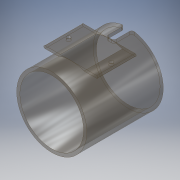
# Autodesk Inventor part: Propeller Shroud
Saved by Autodesk Inventor 2019 (Build 230136000, 136)
## iProperties
Created: 2019-02-08
Part Number: Propeller Shroud
Material: ABS Plastic
Document SubType Name: Modeling
Designer: User
Density: 1.06 g/cm^3
Appearance: Dark Bronze Reflective
Mass: 159.619 g
Surface Area: 631.201 cm^2
Volume: 150.584 cm^3
Author: User
Autodesk Inventor part; units mm, degrees
ref_plane "YZ Plane" through (0, 0, 0) normal (1, 0, 0) x (0, 1, 0)
ref_plane "XZ Plane" through (0, 0, 0) normal (0, 1, 0) x (-1, 0, 0)
ref_plane "XY Plane" through (0, 0, 0) normal (0, 0, 1) x (1, 0, 0)
sketch "Sketch1" plane through (0, 0, 0) normal (0, 0, 1) x (1, 0, 0)
  arc A0 (-20.5913, 51) -> (20.5913, 51) centre (0, 0) ccw
  circle A1 centre (0, 0) radius 50
  line L0 (-40.5, 55) -> (40.5, 55)
  arc A2 (-40.5, 55) -> (-40.5, 51) centre (-40.5, 53) ccw
  arc A3 (40.5, 51) -> (40.5, 55) centre (40.5, 53) ccw
  line L1 (40.5, 51) -> (19.5959, 51)
  line L2 (40.5, 51) -> (19.5959, 51)
  line L3 (40.5, 51) -> (19.5959, 51)
  line L4 (19.5959, 51) -> (-40.5, 51)
  line L5 (0, 51) -> (0, 50)
  dimension "d0" = 110
  dimension "d1" = 100
  constraints: 12 end point, 6 point on circle, 4 centre point, 3 point on line, 2 coincident, 1 horizontal, 1 vertical
  measures "d0" diameter of A0
  measures "d1" diameter of A1
extrude "Extrusion1" add sketch "Sketch1" against normal blind 120
sketch "Sketch2" plane through (0, 0, 0) normal (0, 0, 1) x (1, 0, 0)
  circle A0 centre (0, 0) radius 50 projected
  line L0 (-40.5, 51) -> (-20.5913, 51) projected
  arc A1 (-20.5913, 51) -> (20.5913, 51) centre (0, 0) ccw projected
  line L1 (20.5913, 51) -> (40.5, 51) projected
  arc A2 (40.5, 51) -> (40.5, 55) centre (40.5, 53) ccw projected
  line L2 (40.5, 55) -> (-40.5, 55) projected
  arc A3 (-40.5, 55) -> (-40.5, 51) centre (-40.5, 53) ccw projected
  circle A4 centre (0, 0) radius 55
  point P0 (160.5446, 51)
  constraints: 1 coincident, 3 other
extrude "Extrusion2" cut sketch "Sketch2" against normal blind 30 contours A3 L2 A4 L0 | L2 A2 L1 A4
ref_plane "Work Plane1" through (0, 0, -60) normal (0, 0, 1) x (1, 0, 0)
sketch "Sketch3" plane through (50, 55, 0) normal (0, 1, 0) x (1, 0, 0)
  line L0 (-44, 120) -> (-56, 120)
  line L1 (-30.4041, 0) -> (-69.5959, 0) projected
  line L2 (-56, 120) -> (-44, 120)
  line L3 (-44, 120) -> (-44, 95)
  line L4 (-48, 91) -> (-52, 91)
  line L5 (-56, 95) -> (-56, 120)
  arc A0 (-56, 95) -> (-52, 91) centre (-52, 95) ccw
  arc A1 (-48, 91) -> (-44, 95) centre (-48, 95) ccw
  point P0 (17.7764, 120)
  point P1 (-44, 91)
  point P2 (-56, 91)
  dimension "d33" = 12
  dimension "d43" = 12
  dimension "d44" = 29
  dimension "d45" = 4
  constraints: 10 end point, 4 point on circle, 4 point on line, 4 tangent, 2 centre point, 2 parallel, 1 equal radius, 1 horizontal, 1 perpendicular
  measures "d33" distance of L0.start L0.end
  measures "d43" distance of point (-44, 91) point (-56, 91)
  measures "d44" distance of L2.end point (-44, 91)
  measures "d45" radius of A0
extrude "Extrusion3" cut sketch "Sketch3" against normal blind 7
mirror "Mirror2" about plane through (0, 0, -60) normal (0, 0, 1) of "Extrusion2"
fillet "Fillet1" radius 4 2 edges at (-6, 52.1552, -120) (6, 52.1552, -120)
sketch "Sketch4" plane through (-40.5, 55, -30) normal (0, 1, 0) x (1, 0, 0)
  line L0 (40.5, 60) -> (0, 60) projected
  line L1 (0, 0) -> (0, 60) projected
  line L2 (0, 0) -> (40.5, 0) projected
  line L3 (40.5, 0) -> (81, 0) projected
  line L4 (81, 0) -> (81, 60) projected
  line L5 (81, 60) -> (40.5, 60) projected
  line L6 (81, 0) -> (81, 60) projected
  line L7 (19.9087, 60) -> (19.9087, 0) projected
  line L8 (61.0913, 0) -> (61.0913, 60) projected
  line L9 (81, 0) -> (61.0913, 0) projected
  circle A0 centre (6.9544, 30) radius 3
  circle A1 centre (74.0456, 30) radius 3
  point P0 (40.5, -30)
  dimension "d48" = 6
  dimension "d51" = 6
  constraints: 2 centre point
  measures "d48" diameter of A1
  measures "d51" diameter of A0
extrude "Extrusion4" cut sketch "Sketch4" against normal blind 5 contours A0 | A1
body "Solid1"
